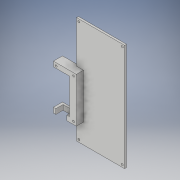
# Autodesk Inventor part: PhoneAndScannerCover
Saved by Autodesk Inventor 2019 (Build 230136000, 136)
## iProperties
Created: 2019-01-25
Part Number: PhoneAndScannerCover
Material: Generic
Document SubType Name: Modeling
Designer: garretthagen21
Density: 1 g/cm^3
Appearance: Default
Author: garretthagen21
Autodesk Inventor part; units mm, degrees
ref_plane "YZ Plane" through (0, 0, 0) normal (1, 0, 0) x (0, 1, 0)
ref_plane "XZ Plane" through (0, 0, 0) normal (0, 1, 0) x (-1, 0, 0)
ref_plane "XY Plane" through (0, 0, 0) normal (0, 0, 1) x (1, 0, 0)
sketch "Sketch1" plane through (0, 0, 0) normal (0, 0, 1) x (1, 0, 0)
  line L0 (10.4417, 4.052) -> (-51.2803, 4.052)
  line L1 (-51.2803, 4.052) -> (-51.2803, -50.05)
  line L2 (-51.2803, -107.708) -> (-51.2803, -133.108)
  line L3 (-51.2803, -133.108) -> (10.4417, -133.108)
  line L4 (10.4417, -133.108) -> (10.4417, 4.052)
  line L5 (-51.2803, -101.358) -> (-51.2803, -56.4)
  line L6 (-51.2803, -50.05) -> (-71.8543, -50.05)
  line L7 (-71.8543, -50.05) -> (-71.8543, -56.4)
  line L8 (-71.8543, -56.4) -> (-51.2803, -56.4)
  line L9 (-51.2803, -107.708) -> (-71.8543, -107.708)
  line L10 (-71.8543, -107.708) -> (-71.8543, -101.358)
  line L11 (-71.8543, -101.358) -> (-51.2803, -101.358)
  point P0 (0, 0)
  dimension "d0" = 61.722
  dimension "d1" = 54.102
  dimension "d4" = 25.4
  dimension "d22" = 20.574
  dimension "d23" = 6.35
  dimension "d24" = 6.35
  constraints: 24 end point, 4 perpendicular, 3 vertical, 2 horizontal, 2 parallel, 2 point on line
  measures "d0" distance of L0.start L0.end
  measures "d1" distance of L0.end L1.end
  measures "d4" distance of L2.start L2.end
  measures "d22" distance of L1.end L6.end
  measures "d23" distance of L6.end L7.end
  measures "d24" distance of L9.end L10.end
extrude "Extrusion1" add sketch "Sketch1" along normal blind 2.54
sketch "Sketch2" plane through (0, 0, 2.54) normal (0, 0, 1) x (1, 0, 0)
  line L0 (10.4417, 4.052) -> (-51.2803, 4.052) projected
  line L1 (-51.2803, 4.052) -> (-51.2803, -133.108) projected
  line L2 (10.4417, -133.108) -> (10.4417, 4.052) projected
  line L3 (-51.2803, -133.108) -> (10.4417, -133.108) projected
  point P0 (0, 0)
  point P1 (-48.2323, 1.004)
  point P2 (7.3937, 1.004)
  point P3 (-48.2323, -130.06)
  point P4 (7.3937, -130.06)
  dimension "d7" = 3.048
  dimension "d8" = 3.048
  dimension "d9" = 3.048
  dimension "d10" = 3.048
  measures "d7" distance from line of L0 point (-48.232, 1.004)
  measures "d8" distance from line of L1 point (-48.232, 1.004)
  measures "d9" distance from line of L2 point (7.394, 1.004)
  measures "d10" distance from line of L3 point (-48.232, -130.06)
hole "Hole1" at (-48.2323, 1.004, 2.54) at (7.3937, 1.004, 2.54) at (-48.2323, -130.06, 2.54) at (7.3937, -130.06, 2.54) direction (0, 0, -1) diameter 2.54 depth 25.4 tip angle 118
sketch "Sketch3" plane through (0, 0, 2.54) normal (0, 0, 1) x (1, 0, 0)
  line L0 (-51.2803, -107.708) -> (-42.3903, -107.708)
  line L1 (-51.2803, -50.05) -> (-42.3903, -50.05)
  line L2 (-42.3903, -50.05) -> (-42.3903, -107.708)
  line L3 (-51.2803, -50.05) -> (-71.8543, -50.05) projected
  line L4 (-71.8543, -56.4) -> (-51.2803, -56.4) projected
  line L5 (-71.8543, -50.05) -> (-51.2803, -50.05)
  line L6 (-51.2803, -56.4) -> (-71.8543, -56.4)
  line L7 (-71.8543, -56.4) -> (-71.8543, -50.05)
  line L8 (-51.2803, -101.358) -> (-71.8543, -101.358) projected
  line L9 (-51.2803, -101.358) -> (-54.4553, -101.358)
  line L10 (-71.8543, -107.708) -> (-51.2803, -107.708) projected
  line L11 (-54.4553, -107.708) -> (-51.2803, -107.708)
  line L12 (-54.4553, -101.358) -> (-54.4553, -107.708)
  line L13 (-71.8543, -101.358) -> (-68.6793, -101.358)
  line L14 (-68.6793, -101.358) -> (-68.6793, -107.708)
  line L15 (-68.6793, -107.708) -> (-71.8543, -107.708)
  line L16 (-71.8543, -107.708) -> (-71.8543, -101.358)
  line L17 (-51.2803, -56.4) -> (-51.2803, -101.358)
  point P0 (0, 0)
  point P1 (-51.2803, 4.052)
  point P2 (-51.2803, -133.108)
  dimension "d25" = 3.175
  dimension "d26" = 3.175
  dimension "d33" = 8.89
  constraints: 28 end point, 3 parallel, 3 point on line, 2 horizontal, 2 perpendicular, 2 vertical, 1 collinear
  measures "d25" distance of L14.end L15.end
  measures "d26" distance of L8.start L9.end
  measures "d33" distance between parallel lines of L2 L17
extrude "Extrusion2" add sketch "Sketch3" along normal blind 9.144 contours L10 L12 L8 L17 L4 L7 L3 L1 L2 L0 | L10 L16 L8 L14
sketch "Sketch4" plane through (0, 0, 11.684) normal (0, 0, 1) x (1, 0, 0)
  line L0 (-42.3903, -50.05) -> (-71.8543, -50.05) projected
  line L1 (-42.3903, -107.708) -> (-42.3903, -50.05) projected
  line L2 (-71.8543, -50.05) -> (-71.8543, -56.4) projected
  line L3 (-54.4553, -107.708) -> (-42.3903, -107.708) projected
  point P0 (0, 0)
  point P1 (-45.9463, -53.606)
  point P2 (-45.9463, -104.152)
  point P3 (-68.2983, -53.606)
  dimension "d29" = 3.556
  dimension "d30" = 3.556
  dimension "d31" = 3.556
  dimension "d32" = 3.556
  dimension "d41" = 3.556
  measures "d29" distance from line of point (-45.946, -53.606) L0
  measures "d30" distance from line of point (-45.946, -53.606) L1
  measures "d31" distance from line of L2 point (-68.298, -53.606)
  measures "d32" distance from line of point (-45.946, -104.152) L3
  measures "d41" distance from line of L1 point (-45.946, -104.152)
hole "Hole2" at (-45.9463, -53.606, 11.684) at (-45.9463, -104.152, 11.684) at (-68.2983, -53.606, 11.684) direction (0, 0, -1) diameter 2.54 depth 4.572 tip angle 118
body "Solid1"
